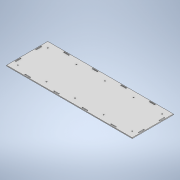
# Autodesk Inventor part: BungaSign-Bigger-Back
Saved by Autodesk Inventor 2022 (Build 260153000, 153)
## iProperties
Created: 2022-08-11
Part Number: BungaSign-Bigger-Back
Material: Generic
Document SubType Name: Modeling
Designer: incep
Density: 1 g/cm^3
Appearance: Default
Author: incep
Autodesk Inventor part; units mm, degrees
ref_plane "YZ Plane" through (0, 0, 0) normal (1, 0, 0) x (0, 1, 0)
ref_plane "XZ Plane" through (0, 0, 0) normal (0, 1, 0) x (-1, 0, 0)
ref_plane "XY Plane" through (0, 0, 0) normal (0, 0, 1) x (1, 0, 0)
sketch "Sketch1" plane through (0, 0, 0) normal (0, 1, 0) x (-1, 0, 0)
  line L0 (254, -152.4) -> (-254, -152.4) construction
  line L1 (-254, -152.4) -> (-254, 152.4) construction
  line L2 (-254, 152.4) -> (254, 152.4) construction
  line L3 (254, 152.4) -> (254, -152.4) construction
  line L4 (250, -150) -> (-250, -150) construction
  line L5 (-250, -150) -> (-250, 150) construction
  line L6 (-250, 150) -> (250, 150) construction
  line L7 (250, 150) -> (250, -150) construction
  line L8 (35, -51) -> (-35, -51) construction
  line L9 (-35, -51) -> (-35, 51) construction
  line L10 (-35, 51) -> (35, 51) construction
  line L11 (35, 51) -> (35, -51) construction
  line L12 (-52, -51) -> (-122, -51) construction
  line L13 (-52, 51) -> (-52, -51) construction
  line L14 (-122, 51) -> (-52, 51) construction
  line L15 (-122, -51) -> (-122, 51) construction
  line L16 (-139, -51) -> (-209, -51) construction
  line L17 (-139, 51) -> (-139, -51) construction
  line L18 (-209, 51) -> (-139, 51) construction
  line L19 (-209, -51) -> (-209, 51) construction
  line L20 (122, -51) -> (52, -51) construction
  line L21 (122, 51) -> (122, -51) construction
  line L22 (52, 51) -> (122, 51) construction
  line L23 (52, -51) -> (52, 51) construction
  line L24 (35, -51) -> (-35, -51) construction
  line L25 (35, 51) -> (35, -51) construction
  line L26 (-35, 51) -> (35, 51) construction
  line L27 (-35, -51) -> (-35, 51) construction
  line L28 (-52, -51) -> (-122, -51) construction
  line L29 (-52, 51) -> (-52, -51) construction
  line L30 (-122, 51) -> (-52, 51) construction
  line L31 (-122, -51) -> (-122, 51) construction
  line L32 (209, -51) -> (139, -51) construction
  line L33 (209, 51) -> (209, -51) construction
  line L34 (139, 51) -> (209, 51) construction
  line L35 (139, -51) -> (139, 51) construction
  line L36 (122, -51) -> (52, -51) construction
  line L37 (122, 51) -> (122, -51) construction
  line L38 (52, 51) -> (122, 51) construction
  line L39 (52, -51) -> (52, 51) construction
  line L40 (35, -51) -> (-35, -51) construction
  line L41 (35, 51) -> (35, -51) construction
  line L42 (-35, 51) -> (35, 51) construction
  line L43 (-35, -51) -> (-35, 51) construction
  line L44 (188.5027, 1.1241) -> (237.2968, 1.1241) construction
  line L45 (194, 27.9543) -> (222.5108, 27.9543) construction
  line L46 (235, -77) -> (-235, -77)
  line L47 (-235, -77) -> (-235, 77)
  line L48 (-235, 77) -> (235, 77)
  line L49 (235, 77) -> (235, -77)
  circle A0 centre (0, -56) radius 1.85
  circle A1 centre (107, -56) radius 1.85
  circle A2 centre (-107, -56) radius 1.85
  circle A3 centre (107, 56) radius 1.85
  circle A4 centre (-107, 56) radius 1.85
  circle A5 centre (0, 56) radius 1.85
  circle A6 centre (214, -56) radius 1.85
  circle A7 centre (214, 56) radius 1.85
  circle A8 centre (-214, 56) radius 1.85
  circle A9 centre (-214, -56) radius 1.85
  line L50 (170.5, -74) -> (150.5, -74)
  line L51 (150.5, -74) -> (150.5, -71)
  line L52 (150.5, -71) -> (170.5, -71)
  line L53 (170.5, -71) -> (170.5, -74)
  line L54 (160.5, -74) -> (160.5, -71) construction
  line L55 (170.5, 71) -> (150.5, 71)
  line L56 (150.5, 71) -> (150.5, 74)
  line L57 (150.5, 74) -> (170.5, 74)
  line L58 (170.5, 74) -> (170.5, 71)
  line L59 (160.5, 71) -> (160.5, 74) construction
  line L60 (43.5, -71) -> (63.5, -71)
  line L61 (43.5, -74) -> (43.5, -71)
  line L62 (63.5, -74) -> (43.5, -74)
  line L63 (53.5, -74) -> (53.5, -71) construction
  line L64 (63.5, -71) -> (63.5, -74)
  line L65 (63.5, 71) -> (43.5, 71)
  line L66 (43.5, 71) -> (43.5, 74)
  line L67 (43.5, 74) -> (63.5, 74)
  line L68 (53.5, 71) -> (53.5, 74) construction
  line L69 (63.5, 74) -> (63.5, 71)
  line L70 (-63.5, -71) -> (-43.5, -71)
  line L71 (-63.5, -74) -> (-63.5, -71)
  line L72 (-43.5, -74) -> (-63.5, -74)
  line L73 (-53.5, -74) -> (-53.5, -71) construction
  line L74 (-43.5, -71) -> (-43.5, -74)
  line L75 (-43.5, 71) -> (-63.5, 71)
  line L76 (-63.5, 71) -> (-63.5, 74)
  line L77 (-63.5, 74) -> (-43.5, 74)
  line L78 (-53.5, 71) -> (-53.5, 74) construction
  line L79 (-43.5, 74) -> (-43.5, 71)
  line L80 (-170.5, -71) -> (-150.5, -71)
  line L81 (-170.5, -74) -> (-170.5, -71)
  line L82 (-150.5, -74) -> (-170.5, -74)
  line L83 (-160.5, -74) -> (-160.5, -71) construction
  line L84 (-150.5, -71) -> (-150.5, -74)
  line L85 (-150.5, 71) -> (-170.5, 71)
  line L86 (-170.5, 71) -> (-170.5, 74)
  line L87 (-170.5, 74) -> (-150.5, 74)
  line L88 (-160.5, 71) -> (-160.5, 74) construction
  line L89 (-150.5, 74) -> (-150.5, 71)
  line L90 (232, -48.5) -> (229, -48.5)
  line L91 (229, -48.5) -> (229, -28.5)
  line L92 (229, -28.5) -> (232, -28.5)
  line L93 (232, -28.5) -> (232, -48.5)
  line L94 (232, -38.5) -> (229, -38.5) construction
  line L95 (232, 28.5) -> (229, 28.5)
  line L96 (229, 28.5) -> (229, 48.5)
  line L97 (229, 48.5) -> (232, 48.5)
  line L98 (232, 48.5) -> (232, 28.5)
  line L99 (232, 38.5) -> (229, 38.5) construction
  line L100 (-229, -48.5) -> (-232, -48.5)
  line L101 (-232, -48.5) -> (-232, -28.5)
  line L102 (-232, -28.5) -> (-229, -28.5)
  line L103 (-229, -28.5) -> (-229, -48.5)
  line L104 (-229, 28.5) -> (-232, 28.5)
  line L105 (-232, 28.5) -> (-232, 48.5)
  line L106 (-232, 48.5) -> (-229, 48.5)
  line L107 (-229, 48.5) -> (-229, 28.5)
  line L108 (-229, -38.5) -> (-232, -38.5) construction
  line L109 (-229, 38.5) -> (-232, 38.5) construction
  point P0 (0, 0)
  point P1 (254, 0)
  point P2 (0, -152.4)
  point P3 (0, -150)
  point P4 (-250, 0)
  point P5 (0, -80)
  point P6 (0, -51)
  point P7 (-35, 0)
  point P8 (-87, -51)
  point P9 (-87, 0)
  point P10 (-122, 0)
  point P11 (-174, -51)
  point P12 (-174, 0)
  point P13 (-209, 0)
  point P14 (87, -51)
  point P15 (87, 0)
  point P16 (52, 0)
  point P17 (0, -51)
  point P18 (0, 0)
  point P19 (-35, 0)
  point P20 (-87, -51)
  point P21 (-87, 0)
  point P22 (-122, 0)
  point P23 (174, -51)
  point P24 (174, 0)
  point P25 (139, 0)
  point P26 (87, -51)
  point P27 (87, 0)
  point P28 (52, 0)
  point P29 (0, -51)
  point P30 (0, 0)
  point P31 (-35, 0)
  point P32 (-7, -51)
  point P33 (-21, -51)
  point P34 (7, 51)
  point P35 (21, 51)
  point P36 (-122, -21)
  point P37 (-122, -36)
  point P38 (-160, 51)
  point P39 (-188, 51)
  point P40 (105, -51)
  point P41 (69, -51)
  point P42 (-235, 0)
  point P43 (0, -77)
  point P44 (139, -27.0457)
  point P45 (139, -12.0457)
  dimension "d0" = 508
  dimension "d1" = 304.8
  dimension "d2" = 500
  dimension "d3" = 300
  dimension "d6" = 70
  dimension "d10" = 87
  dimension "d13" = 87
  dimension "d63" = 470
  dimension "d67" = 154
  dimension "d68" = 418
  dimension "d71" = 3.7
  dimension "d72" = 5
  dimension "d73" = 5
  dimension "d74" = 107
  dimension "d75" = 107
  dimension "d76" = 107
  dimension "d77" = 107
  dimension "d78" = 3
  dimension "d79" = 20
  dimension "d80" = 3
  dimension "d81" = 160.5
  dimension "d82" = 20
  dimension "d83" = 3
  dimension "d84" = 3
  dimension "d87" = 107
  dimension "d92" = 3
  dimension "d93" = 20
  dimension "d94" = 38.5
  dimension "d95" = 3
  dimension "d96" = 3
  dimension "d97" = 20
  dimension "d98" = 3
  dimension "d99" = 38.5
  dimension "d100" = 3
  dimension "d101" = 20
  dimension "d102" = 3
  dimension "d103" = 20
  dimension "d104" = 3
  constraints: 220 end point, 20 midpoint, 20 parallel, 15 horizontal, 12 point on line, 11 horizontal alignment, 11 vertical alignment, 10 centre point, 10 perpendicular, 9 equal radius, 7 collinear, 151 other
  measures "d0" distance of L0.start L0.end
  measures "d1" distance of L2.end L0.start
  measures "d2" distance of L4.start L4.end
  measures "d3" distance of L6.end L4.start
  measures "d6" distance of L8.start L8.end
  measures "d10" distance of point (0, -51) point (-87, -51)
  measures "d13" distance of point (0, -51) point (87, -51)
  measures "d63" distance of L46.start L46.end
  measures "d67" distance of L48.end L46.start
  measures "d68" distance between parallel lines of L19 L33
  measures "d71" diameter of A0
  measures "d72" distance from line of A0.centre L8
  measures "d73" distance from line of L10 A5.centre
  measures "d74" distance of A0.centre A1.centre
  measures "d75" distance of A2.centre A0.centre
  measures "d76" distance of A6.centre A1.centre
  measures "d77" distance of A9.centre A2.centre
  measures "d78" distance between parallel lines of L52 L50
  measures "d79" distance of L50.start L50.end
  measures "d80" distance between parallel lines of L46 L50
  measures "d81" horizontal distance of point (0, -77) L54.start
  measures "d82" distance of L55.start L55.end
  measures "d83" distance of L55.end L56.end
  measures "d84" distance between parallel lines of L48 L57
  measures "d87" distance of L51.end L60.start
  measures "d92" distance of L90.start L90.end
  measures "d93" distance of L90.end L91.end
  measures "d94" vertical distance of point (0, 0) L94.start
  measures "d95" distance between parallel lines of L49 L93
  measures "d96" distance of L95.start L95.end
  measures "d97" distance of L95.end L96.end
  measures "d98" distance between parallel lines of L49 L98
  measures "d99" vertical distance of point (0, 0) L99.start
  measures "d100" distance of L100.start L100.end
  measures "d101" distance of L102.end L100.start
  measures "d102" distance of L104.start L104.end
  measures "d103" distance of L106.end L104.start
  measures "d104" distance between parallel lines of L47 L101
extrude "Extrusion2" add sketch "Sketch1" along normal blind 3
equation "\"thickness\" = 3"
equation "\"kerf\" = 0.1"
equation "\"loose\" = 1.05"
body "Solid2"
